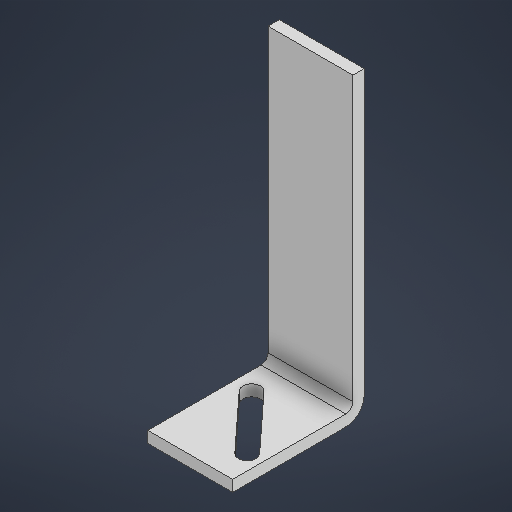
# Autodesk Inventor part: Conveyor mounting bracket
Saved by Autodesk Inventor 2027 (Build 310192000, 192)
## iProperties
Created: 2026-04-16
Part Number: Conveyor mounting bracket
Material: Generic
Document SubType Name: Modeling
Designer: ratik
Density: 1 g/cm^3
Appearance: Default
Author: ratik
Autodesk Inventor part; units mm, degrees
ref_plane "YZ Plane" through (0, 0, 0) normal (1, 0, 0) x (0, 1, 0)
ref_plane "XZ Plane" through (0, 0, 0) normal (0, 1, 0) x (-1, 0, 0)
ref_plane "XY Plane" through (0, 0, 0) normal (0, 0, 1) x (1, 0, 0)
sketch "Sketch1" plane through (0, 0, 0) normal (1, 0, 0) x (0, 1, 0)
  line L0 (108.0556, -3.1511) -> (8.0556, -3.1511)
  line L1 (8.0556, -7.1511) -> (108.0556, -7.1511)
  line L2 (108.0556, -7.1511) -> (108.0556, -3.1511)
  line L3 (5.5556, 39.3489) -> (1.5556, 39.3489)
  line L4 (1.5556, 39.3489) -> (1.5556, -0.6511)
  line L5 (5.5556, -0.6511) -> (5.5556, 39.3489)
  arc A0 (5.5556, -0.6511) -> (8.0556, -3.1511) centre (8.0556, -0.6511) ccw
  arc A1 (1.5556, -0.6511) -> (8.0556, -7.1511) centre (8.0556, -0.6511) ccw
  point P0 (0, 0)
  dimension "d0" = 4
  dimension "d1" = 100
  dimension "d4" = 40
  dimension "d5" = 4
  dimension "d6" = 2.5
  dimension "d10" = 6.5
  constraints: 12 end point, 4 point on circle, 2 centre point, 2 horizontal, 2 parallel, 1 perpendicular
  measures "d0" distance of L1.end L0.start
  measures "d1" distance of L1.start L1.end
  measures "d4" distance of L5.start L3.start
  measures "d5" distance of L3.start L3.end
  measures "d6" radius of A0
  measures "d10" radius of A1
extrude "Extrusion1" add sketch "Sketch1" along normal blind 30
sketch "Sketch2" plane through (0, 5.5556, 39.3489) normal (0, 1, 0) x (1, 0, 0)
  line L0 (8.558, 32.5205) -> (27, 12.5205)
  line L1 (22.442, 8.3175) -> (4, 28.3175)
  line L2 (0, 40) -> (0, 0) projected
  line L3 (30, 40) -> (30, 0) projected
  arc A0 (22.442, 8.3175) -> (27, 12.5205) centre (24.721, 10.419) ccw
  arc A1 (8.558, 32.5205) -> (4, 28.3175) centre (6.279, 30.419) ccw
  point P0 (0, 39.3489)
  dimension "d13" = 20
  dimension "d14" = 4
  dimension "d15" = 3
  dimension "d16" = 6.2
  dimension "d17" = 6.2
  dimension "d18" = 6.2
  constraints: 4 end point, 4 point on circle, 2 centre point, 1 parallel
  measures "d13" vertical distance of L1.start L1.end
  measures "d14" distance from line of L2 L1.end
  measures "d15" distance from line of L3 L0.end
  measures "d16" distance between parallel lines of L1 L0
  measures "d17" diameter of A0
  measures "d18" diameter of A1
extrude "Extrusion2" cut sketch "Sketch2" against normal blind 30
body "Solid1"
